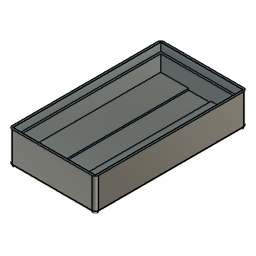
Controller_Bottom v3 (Autodesk Fusion 360 design; units mm, degrees)
Autodesk Fusion 360 part; units mm, degrees
sketch "Sketch1" plane through (0, 0, 0) normal (0, 0, 1) x (1, 0, 0)
  line L0 (-27, -47.5) -> (27, -47.5)
  line L1 (27, -47.5) -> (27, 47.5)
  line L2 (27, 47.5) -> (-27, 47.5)
  line L3 (-27, 47.5) -> (-27, -47.5)
  line L4 (-27, -47.5) -> (27, 47.5) construction
  line L5 (27, -47.5) -> (-27, 47.5) construction
  dimension "d1" = 95
  dimension "d2" = 54
  constraint horizontal L0
  constraint perpendicular L0 L1
  constraint parallel L0 L2
  constraint parallel L1 L3
  constraint coincident L4 origin
  constraint coincident L5 origin
  measures "d1" distance of L0 L2
  measures "d2" distance of L1 L3
extrude "Extrude1" add sketch "Sketch1" along normal blind 11
sketch "Sketch2" plane through (0, 0, 11) normal (0, 0, 1) x (-1, 0, 0)
  line L0 (27, -47.5) -> (27, 47.5)
  line L1 (27, 47.5) -> (-27, 47.5)
  line L2 (-27, 47.5) -> (-27, -47.5)
  line L3 (-27, -47.5) -> (27, -47.5)
  line L4 (24.5, -45) -> (-24.5, -45)
  line L5 (-24.5, -45) -> (-24.5, 45)
  line L6 (-24.5, 45) -> (24.5, 45)
  line L7 (24.5, 45) -> (24.5, -45)
  line L8 (24.5, -45) -> (-24.5, 45) construction
  line L9 (-24.5, -45) -> (24.5, 45) construction
  dimension "d5" = 2.5
  dimension "d6" = 2.5
  dimension "d7" = 2.5
  dimension "d8" = 90
  constraint horizontal L4
  constraint perpendicular L4 L5
  constraint parallel L4 L6
  constraint parallel L5 L7
  constraint coincident L8 origin
  constraint coincident L9 origin
  measures "d5" distance of L3 L4
  measures "d6" distance of L1 L6
  measures "d7" distance of L2 L5
  measures "d8" distance of L4 L6
extrude "Extrude2" add sketch "Sketch2" along normal blind 5
extrude "Extrude3" cut 1 faces at (-8.1667, -15, 11) along direction (0, 0, -1) blind 5
sketch "Sketch3" plane through (0, 0, 6) normal (0, 0, 1) x (-1, 0, 0)
  line L0 (-24.5, 45) -> (-24.5, -45)
  line L1 (-24.5, -45) -> (24.5, -45)
  line L2 (24.5, -45) -> (24.5, 45)
  line L3 (24.5, 45) -> (-24.5, 45)
  line L4 (7, 45) -> (-7, 45)
  line L5 (-7, 45) -> (-7, -45)
  line L6 (-7, -45) -> (7, -45)
  line L7 (7, -45) -> (7, 45)
  line L8 (7, 45) -> (-7, -45) construction
  line L9 (-7, 45) -> (7, -45) construction
  dimension "d13" = 90
  dimension "d14" = 14
  constraint horizontal L4
  constraint perpendicular L4 L5
  constraint parallel L4 L6
  constraint parallel L5 L7
  constraint coincident L8 origin
  constraint coincident L9 origin
  measures "d13" distance of L4 L6
  measures "d14" distance of L5 L7
extrude "Extrude4" add sketch "Sketch3" along normal blind 8 contours L1 L3 L4 L5 L6 L7
sketch "Sketch4" plane through (0, 0, 14) normal (0, 0, 1) x (-1, 0, 0)
  line L0 (7, -45) -> (7, 45)
  line L1 (7, 45) -> (-7, 45)
  line L2 (-7, 45) -> (-7, -45)
  line L3 (-7, -45) -> (7, -45)
  line L4 (-5, 43) -> (5, 43)
  line L5 (5, 43) -> (5, -43)
  line L6 (5, -43) -> (-5, -43)
  line L7 (-5, -43) -> (-5, 43)
  line L8 (-5, 43) -> (5, -43) construction
  line L9 (5, 43) -> (-5, -43) construction
  dimension "d17" = 2
  dimension "d18" = 2
  constraint horizontal L4
  constraint perpendicular L4 L5
  constraint parallel L4 L6
  constraint parallel L5 L7
  constraint coincident L8 origin
  constraint coincident L9 origin
  measures "d17" distance of L2 L7
  measures "d18" distance of L3 L6
extrude "Extrude5" cut sketch "Sketch4" against normal blind 9 contours L4 L5 L6 L7
sketch "Sketch5" plane through (0, 0, 5) normal (0, 0, 1) x (-1, 0, 0)
  line L0 (-5, -43) -> (5, -43)
  line L1 (5, -43) -> (5, 43)
  line L2 (5, 43) -> (-5, 43)
  line L3 (-5, 43) -> (-5, -43)
  line L4 (-1.5, 36.5) -> (1.5, 36.5)
  line L5 (1.5, 36.5) -> (1.5, -36.5)
  line L6 (1.5, -36.5) -> (-1.5, -36.5)
  line L7 (-1.5, -36.5) -> (-1.5, 36.5)
  line L8 (-1.5, 36.5) -> (1.5, -36.5) construction
  line L9 (1.5, 36.5) -> (-1.5, -36.5) construction
  dimension "d21" = 3
  dimension "d22" = 73
  constraint horizontal L4
  constraint perpendicular L4 L5
  constraint parallel L4 L6
  constraint parallel L5 L7
  constraint coincident L8 origin
  constraint coincident L9 origin
  measures "d21" horizontal distance of L4.start L5.end
  measures "d22" distance of L4 L6
extrude "Extrude6" cut sketch "Sketch5" against normal blind 5 contours L4 L5 L6 L7
sketch "Sketch6" plane through (0, 0, 16) normal (0, 0, 1) x (-1, 0, 0)
  line L0 (-24.5, 45) -> (24.5, 45)
  line L1 (24.5, 45) -> (24.5, -45)
  line L2 (24.5, -45) -> (-24.5, -45)
  line L3 (-24.5, -45) -> (-24.5, 45)
  line L4 (-27, -47.5) -> (27, -47.5)
  line L5 (27, -47.5) -> (27, 47.5)
  line L6 (27, 47.5) -> (-27, 47.5)
  line L7 (-27, 47.5) -> (-27, -47.5)
  line L8 (-25.75, -46.25) -> (25.75, -46.25)
  line L9 (25.75, -46.25) -> (25.75, 46.25)
  line L10 (25.75, 46.25) -> (-25.75, 46.25)
  line L11 (-25.75, 46.25) -> (-25.75, -46.25)
  line L12 (-25.75, -46.25) -> (25.75, 46.25) construction
  line L13 (25.75, -46.25) -> (-25.75, 46.25) construction
  dimension "d25" = 1.25
  dimension "d26" = 1.25
  constraint horizontal L8
  constraint perpendicular L8 L9
  constraint parallel L8 L10
  constraint parallel L9 L11
  constraint coincident L12 origin
  constraint coincident L13 origin
  measures "d25" distance of L5 L9
  measures "d26" distance of L6 L10
extrude "Extrude7" add sketch "Sketch6" along normal blind 5 contours L8 L9 L10 L11
sketch "Sketch7" plane through (0, 47.5, 0) normal (0, 1, 0) x (-1, 0, 0)
  line L0 (-27, 0) -> (27, 0)
  line L1 (27, 0) -> (27, 16)
  line L2 (27, 16) -> (-27, 16)
  line L3 (-27, 16) -> (-27, 0)
  circle A0 centre (14.9884, 9.9657) radius 2.5
  dimension "d29" = 5
  measures "d29" diameter of A0
extrude "Extrude18" cut 1 faces at (6.3333, -14.3333, 14) along direction (0, 0, -1) blind 9
extrude "Extrude19" add 1 faces at (-1.5, -12.1667, 3.3333) along direction (1, 0, 0) blind 5
extrude "Extrude20" cut 1 faces at (25.3333, 15, 21) along direction (0, 0, -1) blind 5
sketch "Sketch16" plane through (0, 0, 16) normal (0, 0, 1) x (-1, 0, 0)
  line L0 (24.5, -45) -> (-24.5, -45)
  line L1 (-24.5, -45) -> (-24.5, 45)
  line L2 (-24.5, 45) -> (24.5, 45)
  line L3 (24.5, 45) -> (24.5, -45)
  line L4 (-27, -47.5) -> (27, -47.5)
  line L5 (27, -47.5) -> (27, 47.5)
  line L6 (27, 47.5) -> (-27, 47.5)
  line L7 (-27, 47.5) -> (-27, -47.5)
  line L8 (27, -47.5) -> (-27, -47.5)
  line L9 (-27, -47.5) -> (-27, 47.5)
  line L10 (-27, 47.5) -> (27, 47.5)
  line L11 (27, 47.5) -> (27, -47.5)
  line L12 (27, -47.5) -> (-27, 47.5) construction
  line L13 (-27, -47.5) -> (27, 47.5) construction
  dimension "d66" = 54
  dimension "d67" = 95
  constraint horizontal L8
  constraint perpendicular L8 L9
  constraint parallel L8 L10
  constraint parallel L9 L11
  constraint coincident L12 origin
  constraint coincident L13 origin
  measures "d66" distance of L9 L11
  measures "d67" distance of L8 L10
extrude "Extrude21" add sketch "Sketch16" along normal blind 5
sketch "Sketch17" plane through (0, 0, 21) normal (0, 0, 1) x (-1, 0, 0)
  line L0 (-24.5, 45) -> (24.5, 45)
  line L1 (24.5, 45) -> (24.5, -45)
  line L2 (24.5, -45) -> (-24.5, -45)
  line L3 (-24.5, -45) -> (-24.5, 45)
  line L4 (27, 47.5) -> (-27, 47.5)
  line L5 (-27, 47.5) -> (-27, -47.5)
  line L6 (-27, -47.5) -> (27, -47.5)
  line L7 (27, -47.5) -> (27, 47.5)
sketch "Sketch18" plane through (0, 0, 21) normal (0, 0, 1) x (-1, 0, 0)
  line L0 (25.75, -46.25) -> (-25.75, -46.25)
  line L1 (-25.75, -46.25) -> (-25.75, 46.25)
  line L2 (-25.75, 46.25) -> (25.75, 46.25)
  line L3 (25.75, 46.25) -> (25.75, -46.25)
  line L4 (25.75, -46.25) -> (-25.75, 46.25) construction
  line L5 (-25.75, -46.25) -> (25.75, 46.25) construction
  line L6 (27, -47.5) -> (27, 47.5)
  line L7 (-27, -47.5) -> (27, -47.5)
  dimension "d70" = 1.25
  dimension "d71" = 1.25
  constraint horizontal L0
  constraint perpendicular L0 L1
  constraint parallel L0 L2
  constraint parallel L1 L3
  constraint coincident L4 origin
  constraint coincident L5 origin
  measures "d70" distance of L3 L6
  measures "d71" distance of L0 L7
extrude "Extrude22" cut sketch "Sketch18" against normal blind 5
fillet "Fillet2" radius 2 4 edges at (27, -47.5, 10.5) (-27, -47.5, 10.5) (27, 47.5, 10.5) (-27, 47.5, 10.5)
fillet "Fillet3" radius 2 8 edges at (0, -47.5, 0) (26.4142, -46.9142, 0) (27, 0, 0) (26.4142, 46.9142, 0) (0, 47.5, 0) (-26.4142, 46.9142, 0) (-27, 0, 0) (-26.4142, -46.9142, 0)
sketch "Sketch8" plane through (0, 49.5, 0) normal (0, 1, 0) x (-1, 0, 0)
  circle A0 centre (14.9884, 9.9657) radius 1.5
sketch "Sketch9" plane through (0, 49.5, 0) normal (0, 1, 0) x (-1, 0, 0)
  circle A0 centre (14.9884, 9.9657) radius 1.5
  point P0 (14.9884, 9.9657)
  dimension "d34" = 3
  constraint coincident P0 A0.centre
  measures "d34" diameter of A0
extrude "Extrude9" [suppressed]
sketch "Sketch10" plane through (0, 0, 0) normal (1, 0, 0) x (0, 1, 0)
sketch "Sketch11" plane through (0, 47.5, 0) normal (0, 1, 0) x (-1, 0, 0)
  circle A0 centre (14.9884, 9.9657) radius 2.5
  line L0 (-27, 0) -> (27, 0)
  line L1 (27, 0) -> (27, 16)
  line L2 (27, 16) -> (-27, 16)
  line L3 (-27, 16) -> (-27, 0)
pattern_linear "R-Pattern1" [suppressed]
sketch "Sketch12" plane through (0, 49.5, 0) normal (0, 1, 0) x (-1, 0, 0)
  circle A0 centre (-15.0116, 9.9657) radius 1.5
extrude "Extrude10" [suppressed]
extrude "Extrude11" [suppressed]
sketch "Sketch13" plane through (0, 0, 0) normal (0, 0, -1) x (1, 0, 0)
  line L0 (-1.5, -36.5) -> (-1.5, 36.5)
  line L1 (-1.5, 36.5) -> (1.5, 36.5)
  line L2 (1.5, 36.5) -> (1.5, -36.5)
  line L3 (1.5, -36.5) -> (-1.5, -36.5)
  line L4 (-27, 47.5) -> (-27, -47.5)
  line L5 (-27, -47.5) -> (27, -47.5)
  line L6 (27, -47.5) -> (27, 47.5)
  line L7 (27, 47.5) -> (-27, 47.5)
sketch "Sketch14" plane through (0, 0, 6) normal (0, 0, 1) x (-1, 0, 0)
  line L0 (-7, -45) -> (-7, 45)
  line L1 (-7, 45) -> (-24.5, 45)
  line L2 (-24.5, 45) -> (-24.5, -45)
  line L3 (-24.5, -45) -> (-7, -45)
  line L4 (-9.3113, -19.1689) -> (-21.3113, -19.1689)
  line L5 (-21.3113, -19.1689) -> (-21.3113, -31.1689)
  line L6 (-21.3113, -31.1689) -> (-9.3113, -31.1689)
  line L7 (-9.3113, -31.1689) -> (-9.3113, -19.1689)
  line L8 (-9.3113, -19.1689) -> (-21.3113, -31.1689) construction
  line L9 (-21.3113, -19.1689) -> (-9.3113, -31.1689) construction
  point P0 (-15.3113, -25.1689)
  dimension "d45" = 12
  dimension "d46" = 12
  constraint horizontal L4
  constraint perpendicular L4 L5
  constraint parallel L4 L6
  constraint parallel L5 L7
  constraint coincident L8 P0
  constraint coincident L9 P0
  measures "d45" distance of L4 L6
  measures "d46" distance of L5 L7
extrude "Extrude12" [suppressed]
sketch "Sketch15" plane through (0, 0, 2) normal (0, 0, 1) x (-1, 0, 0)
  line L0 (-9.3113, -31.1689) -> (-9.3113, -19.1689)
  line L1 (-9.3113, -19.1689) -> (-21.3113, -19.1689)
  line L2 (-21.3113, -19.1689) -> (-21.3113, -31.1689)
  line L3 (-21.3113, -31.1689) -> (-9.3113, -31.1689)
  circle A0 centre (-15.3113, -25.1689) radius 5.5
  dimension "d49" = 11
  measures "d49" diameter of A0
extrude "Extrude13" [suppressed]
extrude "Extrude14" [suppressed]
extrude "Extrude15" [suppressed]
extrude "Extrude16" [suppressed]
extrude "Extrude17" [suppressed]
